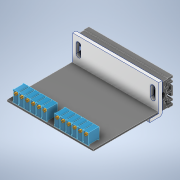
# Autodesk Inventor part: Control Board
Saved by Autodesk Inventor 2021 (Build 250183000, 183)
## iProperties
Created: 2021-04-06
Part Number: Control Board
Material: Generic
Document SubType Name: Modeling
Designer: Andrew
Density: 1 g/cm^3
Appearance: Default
Author: Andrew
Autodesk Inventor part; units mm, degrees
ref_plane "YZ Plane" through (0, 0, 0) normal (1, 0, 0) x (0, 1, 0)
ref_plane "XZ Plane" through (0, 0, 0) normal (0, 1, 0) x (-1, 0, 0)
sketch "Sketch1" plane through (0, 0, 0) normal (1, 0, 0) x (0, 1, 0)
  line L0 (0, 0) -> (24, 0)
  line L1 (24, 0) -> (24, -3)
  line L2 (24, -3) -> (-3, -3)
  line L3 (-3, -3) -> (-3, 8)
  line L4 (-3, 8) -> (0, 8)
  line L5 (0, 8) -> (0, 0)
  line L6 (0, 0) -> (-1, 0)
  line L7 (-1, 0) -> (-1, -3)
  dimension "d0" = 3
  dimension "d1" = 3
  dimension "d2" = 2
  dimension "d3" = 11
  dimension "d4" = 27
  constraints: 16 end point, 6 perpendicular, 2 horizontal, 1 point on line
  measures "d0" distance of L0.end L1.end
  measures "d1" distance of L3.end L4.end
  measures "d2" distance between parallel lines of L3 L7
  measures "d3" distance between parallel lines of L2 L4
  measures "d4" distance of L1.end L2.end
extrude "Extrusion1" add sketch "Sketch1" along normal mid plane 77
extrude "Extrusion2" cut sketch "Sketch1" against normal mid plane 61 contours L6 L7 L2 L3 L4 L5
fillet "Fillet1" radius 2 2 edges at (34.5, -3, -3) (-34.5, -3, -3)
sketch "Sketch2" plane through (0, 0, 0) normal (0, 1, 0) x (-1, 0, 0)
  line L0 (38.5, 58.5) -> (-38.5, 58.5)
  line L1 (-38.5, 58.5) -> (-38.5, 0.5)
  line L2 (-38.5, 0.5) -> (38.5, 0.5)
  line L3 (38.5, 0.5) -> (38.5, 58.5)
  line L4 (38.5, 58.5) -> (-38.5, 0.5) construction
  line L5 (-38.5, 58.5) -> (38.5, 0.5) construction
  line L6 (38.5, 0) -> (-38.5, 0) projected
  point P0 (0, 0)
  point P1 (0, 29.5)
  point P2 (0, 29.5)
  dimension "d10" = 0.5
  dimension "d11" = 58
  constraints: 12 end point, 3 midpoint, 2 parallel, 1 horizontal, 1 perpendicular, 1 point on line, 1 vertical alignment
  measures "d10" distance between parallel lines of L6 L2
  measures "d11" distance of L0.end L1.end
extrude "Extrusion3" add sketch "Sketch2" along normal blind 1.57 separate body
ref_plane "Work Plane1" through (-38.5, 0, 58) normal (0, 0, 1) x (1, 0, 0)
sketch "Sketch3" plane through (-38.5, 0, 58) normal (0, 0, 1) x (1, 0, 0)
  line L0 (4.5, 11.57) -> (9.3, 11.57)
  line L1 (9.3, 11.57) -> (9.3, 1.57)
  line L2 (9.3, 1.57) -> (4.5, 1.57)
  line L3 (4.5, 1.57) -> (4.5, 11.57)
  circle A0 centre (8.05, 10.32) radius 1.175
  line L4 (77, 1.57) -> (0, 1.57) projected
  line L5 (0, 1.57) -> (77, 1.57) construction
  line L6 (0, 1.57) -> (77, 1.57) projected
  line L7 (0, 0) -> (0, 1.57) projected
  line L8 (7.3959, 9.3124) -> (9.0576, 10.9741)
  line L9 (9.0576, 10.9741) -> (8.7041, 11.3276)
  line L10 (8.7041, 11.3276) -> (7.0424, 9.6659)
  line L11 (7.0424, 9.6659) -> (7.3959, 9.3124)
  line L12 (7.3959, 9.3124) -> (8.7041, 11.3276) construction
  line L13 (9.0576, 10.9741) -> (7.0424, 9.6659) construction
  point P0 (38.5, 0)
  point P1 (7.0614, 9.685)
  point P2 (8.685, 11.3086)
  point P3 (9.0386, 10.955)
  point P4 (7.415, 9.3314)
  dimension "d15" = 4.8
  dimension "d16" = 10
  dimension "d17" = 4.5
  dimension "d18" = 2.35
  dimension "d19" = 1.25
  dimension "d20" = 1.25
  dimension "d23" = 0.5
  dimension "d24" = 45
  constraints: 20 end point, 4 parallel, 2 midpoint, 2 perpendicular, 1 centre point, 1 collinear, 1 horizontal, 1 tangent
  measures "d15" distance of L0.start L0.end
  measures "d16" distance of L0.end L1.end
  measures "d17" distance between parallel lines of L7 L3
  measures "d18" diameter of A0
  measures "d19" distance from line of L0 A0.centre
  measures "d20" distance from line of L1 A0.centre
  measures "d23" distance of L8.end L9.end
  measures "d24" angle of L0 L10
extrude "Extrusion4" add sketch "Sketch3" against normal blind 9.5 separate body contours L0 L1 L2 L3 | A0 L8 | L8 A0 L10 | A0 L9 L8 | L8 L11 A0 | A0 L10 L9 | L11 L10 A0 | L10 A0
sketch "Sketch4" plane through (-34, 1.57, 58) normal (-1, 0, 0) x (0, 0, 1)
  line L0 (0, 10) -> (0, 0) projected
  line L1 (0, 10) -> (-9.5, 10) projected
  line L2 (-9.5, 0) -> (-9.5, 10) projected
  line L3 (0, 0) -> (-9.5, 0) projected
  line L4 (-9.5, 10) -> (-8.75, 10)
  line L5 (-8.75, 10) -> (-8.75, 9)
  line L6 (-8.75, 9) -> (-9.5, 9)
  line L7 (-9.5, 9) -> (-9.5, 10)
  line L8 (0, 10) -> (-9.5, 10) projected
  line L9 (0, 10) -> (-0.75, 10)
  line L10 (-0.75, 10) -> (-0.75, 9)
  line L11 (-0.75, 9) -> (0, 9)
  line L12 (0, 9) -> (0, 10)
  line L13 (-9.5, 0) -> (-8.75, 0)
  line L14 (-8.75, 0) -> (-8.75, 1)
  line L15 (-8.75, 1) -> (-9.5, 1)
  line L16 (-9.5, 1) -> (-9.5, 0)
  line L17 (0, 0) -> (-0.75, 0)
  line L18 (-0.75, 0) -> (-0.75, 1)
  line L19 (-0.75, 1) -> (0, 1)
  line L20 (0, 1) -> (0, 0)
  line L21 (-8.75, 0.75) -> (-0.75, 0.75)
  line L22 (-0.75, 0.75) -> (-0.75, 0)
  line L23 (-0.75, 0) -> (-8.75, 0)
  line L24 (-8.75, 0) -> (-8.75, 0.75)
  point P0 (-58, -1.57)
  point P1 (-0.75, 0.75)
  point P2 (0, 1)
  point P3 (0, 9)
  point P4 (-0.75, 10)
  point P5 (-8.75, 10)
  point P6 (-9.5, 9)
  point P7 (-9.5, 1)
  point P8 (-0.75, 0)
  dimension "d32" = 1
  dimension "d33" = 0.75
  dimension "d34" = 0.75
  dimension "d35" = 1
  dimension "d36" = 0.75
  constraints: 40 end point, 10 parallel, 5 horizontal, 5 perpendicular, 5 point on line
  measures "d32" distance of L4.end L5.end
  measures "d33" distance of L5.end L6.end
  measures "d34" distance of L10.end L11.end
  measures "d35" distance of L13.end L14.end
  measures "d36" distance between parallel lines of L23 L21
extrude "Extrusion7" cut sketch "Sketch4" against normal blind 0.5 contours L0 L19 L18 L21 L14 L15 L2 L6 L5 L1 L10 L11 bodies 3
extrude "Extrusion8" cut sketch "Sketch4" against normal through all contours L3 L14 L21 L18 bodies 3
extrude "Extrusion5" add sketch "Sketch3" along normal blind 1.5 separate body contours A0 L8 | L10 A0
extrude "Extrusion6" add sketch "Sketch3" along normal blind 0.5 contours L8 A0 L10 bodies 4
pattern_linear "Rectangular Pattern1" count 6 spacing 5.15 along (1, 0, 0) bodies 3 4
pattern_linear "Rectangular Pattern2" count 2 spacing 37 along (1, 0, 0) bodies 3 4
sketch "Heatsink Mount" plane through (-38.5, 24, 0) normal (0, 0, 1) x (1, 0, 0)
  line L0 (71.75, -6.5) -> (71.75, -14.5) construction
  line L1 (69.6, -6.5) -> (69.6, -14.5)
  line L2 (73.9, -14.5) -> (73.9, -6.5)
  arc A0 (73.9, -6.5) -> (69.6, -6.5) centre (71.75, -6.5) ccw
  arc A1 (69.6, -14.5) -> (73.9, -14.5) centre (71.75, -14.5) ccw
  line L3 (77, 0) -> (77, -24) projected
  line L4 (0, 0) -> (77, 0) projected
  point P0 (38.5, -24)
  point P1 (71.75, -10.5)
  dimension "d44" = 8
  dimension "d45" = 4.3
  dimension "d47" = 6.5
  dimension "d78" = 33.25
  constraints: 8 end point, 4 point on circle, 4 tangent, 2 centre point, 1 midpoint, 1 parallel, 1 vertical
  measures "d44" distance of L0.end L0.start
  measures "d45" distance between parallel lines of L2 L1
  measures "d47" distance from line of L4 L0.start
  measures "d78" distance from line of point (38.5, -24) L0
extrude "Extrusion9" add sketch "Heatsink Mount" against normal up to surface (3 mm away) separate body
mirror "Mirror1" about plane through (0, 0, 0) normal (1, 0, 0) bodies 5
combine bodies "Combine1" operation type subtract main body 1 bodies to subtract 5
sketch "Sketch6" plane through (0, 0, 0) normal (1, 0, 0) x (0, 1, 0)
  line L0 (8.1, -3.5) -> (-0.45, -3.5)
  line L1 (-0.45, -3.5) -> (-0.45, -9.15)
  line L2 (-0.45, -9.15) -> (-1, -9.15)
  line L3 (-1, -9.15) -> (-1, -13.5)
  line L4 (-1, -13.5) -> (0.85, -13.5)
  line L5 (0.85, -13.5) -> (0.85, -7.5)
  line L6 (0.85, -7.5) -> (4.05, -7.5)
  line L7 (4.05, -7.5) -> (4.05, -6.5)
  line L8 (4.05, -6.5) -> (5.85, -6.5)
  line L9 (5.85, -6.5) -> (5.85, -9.05)
  line L10 (5.85, -9.05) -> (3, -9.05)
  line L11 (3, -9.05) -> (3, -13.5)
  line L12 (3, -13.5) -> (4.5, -13.5)
  line L13 (4.5, -13.5) -> (4.5, -10.45)
  line L14 (4.5, -10.45) -> (5.85, -10.45)
  line L15 (5.85, -10.45) -> (7.75, -9.05)
  line L16 (7.75, -9.05) -> (7.75, -8.25)
  line L17 (7.75, -8.25) -> (9.975, -8.25)
  line L18 (9.975, -8.25) -> (9.975, -12.05)
  line L19 (9.975, -12.05) -> (6.8, -12.05)
  line L20 (6.8, -12.05) -> (6.8, -13.5)
  line L21 (6.8, -13.5) -> (10.725, -13.5)
  line L22 (10.725, -13.5) -> (10.725, -6.65)
  line L23 (10.725, -6.65) -> (9.3885, -6.65)
  line L24 (8.1, -3.5) -> (6.6734, -4.9017) construction
  arc A0 (8.1, -3.5) -> (9.3885, -6.65) centre (9.3885, -4.8115) ccw
  line L25 (-1, 0) -> (-1, -3) projected
  point P0 (0, 0)
  dimension "d50" = 2
  dimension "d51" = 10
  dimension "d52" = 1.85
  dimension "d53" = 1.3
  dimension "d54" = 11.175
  dimension "d55" = 4.5
  dimension "d56" = 1.5
  dimension "d57" = 5.5
  dimension "d59" = 1.9
  dimension "d60" = 8.75
  dimension "d61" = 0.75
  dimension "d62" = 7.8
  dimension "d63" = 1.6
  dimension "d64" = 6.85
  dimension "d66" = 1.45
  dimension "d67" = 4.45
  dimension "d68" = 4.35
  dimension "d69" = 6
  dimension "d70" = 3
  dimension "d71" = 1.4
  dimension "d72" = 8.55
  dimension "d73" = 3.175
  dimension "d74" = 0.5
  constraints: 50 end point, 15 perpendicular, 4 point on line, 2 collinear, 2 horizontal, 2 parallel, 2 point on circle, 2 tangent, 2 vertical, 1 centre point
  measures "d50" distance of L0.start L24.end
  measures "d51" distance between parallel lines of L4 L0
  measures "d52" distance of L3.end L4.end
  measures "d53" distance between parallel lines of L1 L5
  measures "d54" distance between parallel lines of L1 L22
  measures "d55" distance between parallel lines of L1 L7
  measures "d56" distance of L11.end L12.end
  measures "d57" distance between parallel lines of L3 L13
  measures "d59" distance between parallel lines of L9 L16
  measures "d60" distance between parallel lines of L3 L16
  measures "d61" distance between parallel lines of L18 L22
  measures "d62" distance between parallel lines of L3 L20
  measures "d63" distance between parallel lines of L23 L17
  measures "d64" distance of L21.end L22.end
  measures "d66" distance of L19.end L20.end
  measures "d67" distance between parallel lines of L12 L10
  measures "d68" distance of L2.end L3.end
  measures "d69" distance of L4.end L5.end
  measures "d70" distance between parallel lines of L0 L8
  measures "d71" distance between parallel lines of L14 L10
  measures "d72" distance of L0.start L0.end
  measures "d74" distance from line of L25.end L0
extrude "Extrusion10" add sketch "Sketch6" along normal mid plane 75 separate body
mirror "Mirror2" about plane through (0, 10.725, -13.5) normal (0, 1, 0) bodies 6
body "Solid1"
body "Solid2"
body "Solid3"
body "Solid4"
